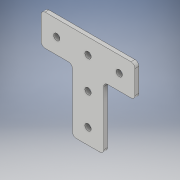
# Autodesk Inventor part: 0.125 T-Gusset
Saved by Autodesk Inventor 2018 (Build 220112000, 112)
## iProperties
Created: 2018-12-30
Part Number: 0.125 T-Gusset
Material: Generic
Document SubType Name: Modeling
Designer: maste
Density: 1 g/cm^3
Appearance: Default
Author: maste
Autodesk Inventor part; units mm, degrees
ref_plane "YZ Plane" through (0, 0, 0) normal (1, 0, 0) x (0, 1, 0)
ref_plane "XZ Plane" through (0, 0, 0) normal (0, 1, 0) x (-1, 0, 0)
ref_plane "XY Plane" through (0, 0, 0) normal (0, 0, 1) x (1, 0, 0)
sketch "Sketch1" plane through (0, 0, 0) normal (0, 0, 1) x (1, 0, 0)
  line L0 (0, 0) -> (25.4, 0)
  line L1 (25.4, 0) -> (25.4, 76.2)
  line L2 (25.4, 76.2) -> (0, 76.2)
  line L3 (0, 76.2) -> (0, 0)
  line L4 (25.4, 76.2) -> (50.8, 76.2)
  line L5 (50.8, 76.2) -> (50.8, 50.8)
  line L6 (50.8, 50.8) -> (25.4, 50.8)
  line L7 (25.4, 50.8) -> (25.4, 76.2)
  line L8 (0, 76.2) -> (-25.4, 76.2)
  line L9 (-25.4, 76.2) -> (-25.4, 50.8)
  line L10 (-25.4, 50.8) -> (0, 50.8)
  line L11 (0, 50.8) -> (0, 76.2)
  dimension "d0" = 25.4
  dimension "d1" = 76.2
  dimension "d2" = 25.4
  dimension "d3" = 25.4
  dimension "d4" = 25.4
  dimension "d5" = 25.4
  constraints: 24 end point, 6 parallel, 3 horizontal, 3 perpendicular
  measures "d0" distance of L2.end L1.end
  measures "d1" distance of L1.end L0.end
  measures "d2" distance of L5.end L6.end
  measures "d3" distance of L4.end L5.end
  measures "d4" distance of L10.end L9.end
  measures "d5" distance of L9.end L8.end
extrude "Extrusion1" add sketch "Sketch1" along normal blind 3.175
sketch "Sketch2" plane through (0, 0, 3.175) normal (0, 0, 1) x (1, 0, 0)
  line L0 (-25.4, 76.2) -> (-25.4, 50.8) construction
  line L1 (-25.4, 63.5) -> (-12.7, 63.5) construction
  line L2 (-12.7, 63.5) -> (12.7, 63.5) construction
  line L3 (12.7, 63.5) -> (38.1, 63.5) construction
  line L4 (12.7, 63.5) -> (12.7, 38.1) construction
  line L5 (12.7, 38.1) -> (12.7, 12.7) construction
  circle A0 centre (-12.7, 63.5) radius 2.5797
  circle A1 centre (12.7, 63.5) radius 2.5797
  circle A2 centre (38.1, 63.5) radius 2.5797
  circle A3 centre (12.7, 38.1) radius 2.5797
  circle A4 centre (12.7, 12.7) radius 2.5797
  point P0 (0, 0)
  dimension "d8" = 12.7
  dimension "d9" = 25.4
  dimension "d10" = 25.4
  dimension "d11" = 25.4
  dimension "d12" = 25.4
  dimension "d13" = 5.1594
  constraints: 10 end point, 5 centre point, 5 coincident, 3 point on line, 1 horizontal, 1 midpoint, 1 vertical
  measures "d8" distance of L1.start L1.end
  measures "d9" distance of L1.end L2.end
  measures "d10" distance of L2.end L3.end
  measures "d11" distance of L2.end L4.end
  measures "d12" distance of L4.end L5.end
  measures "d13" diameter of A0
extrude "Extrusion2" cut sketch "Sketch2" against normal blind 3.175
fillet "Fillet1" radius 3.175 8 edges at (50.8, 76.2, 1.5875) (50.8, 50.8, 1.5875) (25.4, 50.8, 1.5875) (25.4, 0, 1.5875) (0, 0, 1.5875) (0, 50.8, 1.5875) (-25.4, 50.8, 1.5875) (-25.4, 76.2, 1.5875)
body "Solid1"
